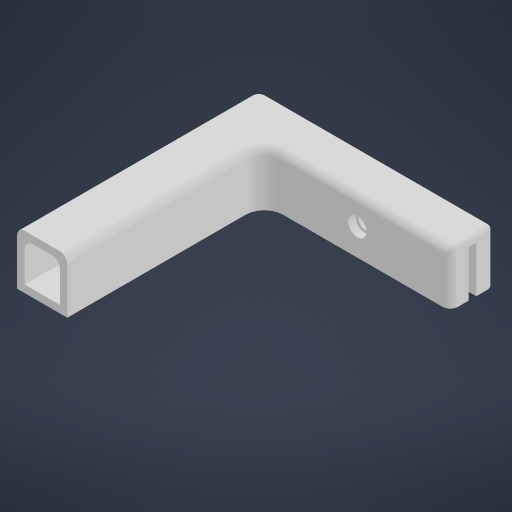
# Autodesk Inventor part: Rod
Saved by Autodesk Inventor 2024.1 (Build 281209000, 209)
## iProperties
Created: 2023-09-06
Part Number: Rod
Material: Generic
Document SubType Name: Modeling
Designer: User
Density: 1 g/cm^3
Appearance: Default
Author: User
Autodesk Inventor part; units mm, degrees
ref_plane "YZ Plane" through (0, 0, 0) normal (1, 0, 0) x (0, 1, 0)
ref_plane "XZ Plane" through (0, 0, 0) normal (0, 1, 0) x (-1, 0, 0)
ref_plane "XY Plane" through (0, 0, 0) normal (0, 0, 1) x (1, 0, 0)
sketch "Sketch1" plane through (0, 0, 0) normal (0, 0, 1) x (1, 0, 0)
  line L0 (0, 0) -> (-13.5, 0)
  line L1 (-13.5, 0) -> (-13.5, 14.5)
  line L2 (-13.5, 14.5) -> (0, 14.5)
  line L3 (0, 14.5) -> (0, 0)
  dimension "d0" = 13.5
  dimension "d1" = 14.5
  constraints: 8 end point, 2 parallel, 1 horizontal, 1 perpendicular
  measures "d0" distance of L1.end L2.end
  measures "d1" distance of L0.end L1.end
extrude "Extrusion1" add sketch "Sketch1" along normal blind 15 and the other way blind 50
sketch "Sketch2" plane through (0, 0, 15) normal (0, 0, 1) x (1, 0, 0)
  line L0 (-13.5, 14.5) -> (-13.5, 0) projected
  line L1 (-13.5, 0) -> (-11.5, 0)
  line L2 (-11.5, 0) -> (-11.5, 2)
  line L3 (-11.5, 2) -> (-13.5, 2)
  line L4 (-13.5, 2) -> (-13.5, 0)
  line L5 (0, 14.5) -> (-13.5, 14.5) projected
  line L6 (0, 14.5) -> (-2, 14.5)
  line L7 (-2, 14.5) -> (-2, 12.5)
  line L8 (-2, 12.5) -> (0, 12.5)
  line L9 (0, 12.5) -> (0, 14.5)
  line L10 (-11.5, 2) -> (-2, 2)
  line L11 (-2, 2) -> (-2, 12.5)
  line L12 (-2, 12.5) -> (-11.5, 12.5)
  line L13 (-11.5, 12.5) -> (-11.5, 2)
  point P0 (0, 0)
  dimension "d4" = 2
  dimension "d5" = 2
  dimension "d6" = 2
  dimension "d7" = 2
  constraints: 24 end point, 6 parallel, 3 horizontal, 3 perpendicular
  measures "d4" distance of L3.end L2.end
  measures "d5" distance of L2.end L1.end
  measures "d6" distance of L8.end L7.end
  measures "d7" distance of L7.end L6.end
extrude "Extrusion2" cut sketch "Sketch2" against normal blind 10 contours L13 L12 L11 L10
fillet "Fillet1" radius 2 2 edges at (-11.5, 12.5, 10) (-2, 12.5, 10)
sketch "Sketch5" plane through (0, 0, 15) normal (1, 0, 0) x (0, 0, -1)
  line L0 (65, 14.5) -> (0, 14.5) projected
  line L1 (65, 14.5) -> (53, 14.5)
  line L2 (53, 14.5) -> (53, 0)
  line L3 (53, 0) -> (65, 0)
  line L4 (65, 0) -> (65, 14.5)
  point P0 (15, 0)
  point P1 (53, 14.5)
  dimension "d14" = 12
  dimension "d15" = 14.5
  constraints: 8 end point, 2 parallel, 1 horizontal, 1 perpendicular
  measures "d14" distance of L3.end L2.end
  measures "d15" distance of L2.end L1.end
extrude "Extrusion3" add sketch "Sketch5" along normal blind 50
sketch "Sketch6" plane through (50, 0, 15) normal (1, 0, 0) x (0, 0, -1)
  line L0 (65, 0) -> (65, 14.5) projected
  line L1 (65, 0) -> (60, 0)
  line L2 (65, 0) -> (70, 0) construction
  line L3 (60, 0) -> (60, 2)
  line L4 (65, 0) -> (0, 0) projected
  line L5 (60, 0) -> (62, 0) construction
  line L6 (65, 14.5) -> (0, 14.5) projected
  line L7 (60, 14.5) -> (60, 12.5)
  line L8 (60, 14.5) -> (62, 14.5) construction
  line L9 (60, 12.5) -> (58, 12.5)
  line L10 (58, 12.5) -> (58, -2.5)
  line L11 (58, -2.5) -> (60, -2.5)
  line L12 (60, -2.5) -> (60, 12.5)
  point P0 (15, 0)
  point P1 (58, 0)
  dimension "d18" = 5
  dimension "d19" = 180
  dimension "d20" = 2
  dimension "d21" = 90
  dimension "d22" = 2
  dimension "d23" = 90
  dimension "d24" = 2
  dimension "d25" = 15
  constraints: 20 end point, 5 horizontal, 3 equal length, 3 perpendicular, 2 parallel, 1 point on line
  measures "d18" distance of L0.start L1.end
  measures "d19" angle of L1 L2
  measures "d20" distance of L1.end L3.end
  measures "d21" angle of L5 L3
  measures "d22" distance of L7.start L7.end
  measures "d23" angle of L7 L8
  measures "d24" distance of L11.end L10.end
  measures "d25" distance of L10.end L9.end
extrude "Extrusion4" cut sketch "Sketch6" against normal blind 50 contours L4 L10 L9 L12 L3 | L12 L11 L10 L4
sketch "Sketch7" plane through (0, 0, -38) normal (0, 0, 1) x (1, 0, 0)
  point P0 (0, 0)
  point P1 (25, 7.25)
hole "Hole1" at (25, 7.25, -38) direction (0, 0, -1) diameter 3.5 depth 7 counterbore diameter 5 counterbore depth 2
fillet "Fillet3" radius 5 1 edges at (0, 7.25, -38)
fillet "Fillet4" radius 2 8 edges at (-13.5, 7.25, -50) (1.4645, 14.5, -36.5355) (27.5, 14.5, -38) (0, 14.5, -9) (-13.5, 14.5, -17.5) (18.25, 14.5, -50) (50, 7.25, -38) (50, 7.25, -50)
fillet "Fillet5" radius 1 3 edges at (50, 14.5, -44) (49.4142, 13.9142, -49.4142) (49.4142, 13.9142, -38.5858)
body "Solid1"
